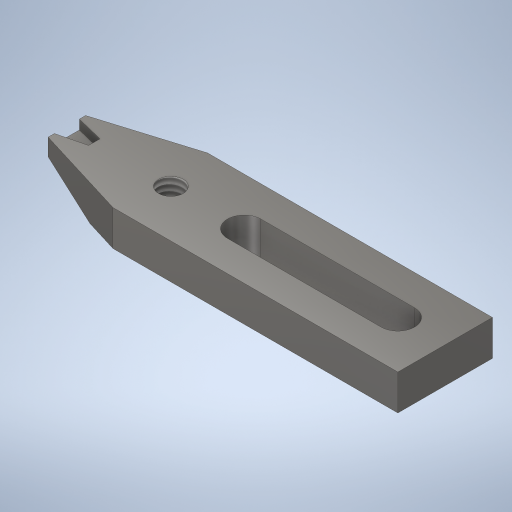
# Autodesk Inventor part: ArmBar-V03- Axel lab
Saved by Autodesk Inventor 2024 (Build 280153000, 153)
## iProperties
Created: 2018-09-07
Part Number: ArmBar-V03- Axel lab
Material: Stainless Steel
Document SubType Name: Modeling
Designer: Tanya
Density: 8 g/cm^3
Appearance: Semi-Polished
Author: Tanya
Autodesk Inventor part; units mm, degrees
ref_plane "YZ Plane" through (0, 0, 0) normal (1, 0, 0) x (0, 1, 0)
ref_plane "XZ Plane" through (0, 0, 0) normal (0, 1, 0) x (-1, 0, 0)
ref_plane "XY Plane" through (0, 0, 0) normal (0, 0, 1) x (1, 0, 0)
sketch "Sketch1" plane through (0, 0, 0) normal (0, 1, 0) x (-1, 0, 0)
  line L0 (0, -8.89) -> (0, 8.89) projected
  line L1 (-35.56, 0) -> (35.56, 0) projected
  line L2 (25.4, -6.35) -> (-25.4, -6.35)
  line L3 (-25.4, -6.35) -> (-25.4, 6.35)
  line L4 (-25.4, 6.35) -> (25.4, 6.35)
  line L5 (25.4, 6.35) -> (25.4, -6.35)
  point P0 (0, 0)
  dimension "d0" = 12.7
  dimension "d1" = 6.35
  dimension "d2" = 50.8
  dimension "d3" = 25.4
  constraints: 8 end point, 2 parallel, 1 horizontal, 1 perpendicular
  measures "d0" distance of L2.end L3.end
  measures "d1" distance between parallel lines of L1 L2
  measures "d2" distance of L2.start L2.end
  measures "d3" distance between parallel lines of L0 L5
extrude "Extrusion1" add sketch "Sketch1" along normal blind 4.7625
sketch "Sketch2" plane through (0, 4.7625, 0) normal (0, 1, 0) x (1, 0, 0)
  line L0 (25.4, 6.35) -> (-25.4, 6.35) projected
  line L1 (-25.4, 6.35) -> (-25.4, -6.35) projected
  line L2 (-25.4, -6.35) -> (25.4, -6.35) projected
  line L3 (25.4, -6.35) -> (25.4, 6.35) projected
  line L4 (-25.4, 2.5146) -> (-12.855, 6.35)
  line L5 (25.4, 6.35) -> (-25.4, 6.35) projected
  line L6 (-25.4, 6.35) -> (-25.4, -6.35) projected
  line L7 (-25.4, -2.5146) -> (-12.855, -6.35)
  line L8 (-12.855, 6.35) -> (-12.855, -6.35) construction
  line L9 (0, 8.89) -> (0, -8.89) projected
  line L10 (35.56, 0) -> (-35.56, 0) projected
  line L11 (-1.5875, 2.2479) -> (19.05, 2.2479)
  line L12 (19.05, 2.2479) -> (19.05, -2.2479)
  line L13 (19.05, -2.2479) -> (-1.5875, -2.2479)
  line L14 (-1.5875, -2.2479) -> (-1.5875, 2.2479)
  circle A0 centre (19.05, 0) radius 2.2479
  circle A1 centre (-1.5875, 0) radius 2.2479
  point P0 (0, 0)
  dimension "d6" = 163
  dimension "d7" = 163
  dimension "d8" = 5.0292
  dimension "d9" = 4.4958
  dimension "d10" = 6.35
  dimension "d11" = 20.6375
  constraints: 14 end point, 7 point on line, 3 parallel, 2 midpoint, 1 centre point, 1 horizontal, 1 perpendicular, 1 tangent, 1 vertical alignment, 2 other
  measures "d6" angle of L0 L4
  measures "d7" angle of L2 L7
  measures "d8" distance of L7.start L4.start
  measures "d9" distance between parallel lines of L13 L11
  measures "d10" distance between parallel lines of L12 L3
  measures "d11" distance of L11.start L11.end
extrude "Extrusion2" cut sketch "Sketch2" against normal through all contours L4 L1 L0 | L11 A0 L10 A1 L9 | L9 A1 L11 | A1 L10 L9 | L9 L10 L14 A1 | L14 L10 A1 | A0 L10 L12 | L12 L10 A0 | L7 L2 L1 | L10 L14 A1 | A0 L12 L10 | L10 A1 L9 | L9 A1 L14 L10 | L10 A0 L13 L9 A1 | L12 A0 L10 | A1 L9 L13
sketch "Sketch3" plane through (0, 4.7625, 0) normal (0, 1, 0) x (1, 0, 0)
  line L0 (-25.4, -2.5146) -> (-12.855, -6.35) projected
  line L1 (-12.855, -6.35) -> (25.4, -6.35) projected
  line L2 (25.4, -6.35) -> (25.4, 6.35) projected
  line L3 (25.4, 6.35) -> (-12.855, 6.35) projected
  line L4 (-12.855, 6.35) -> (-25.4, 2.5146) projected
  line L5 (-25.4, 2.5146) -> (-25.4, -2.5146) projected
  line L6 (19.05, -2.2479) -> (-1.5875, -2.2479) projected
  arc A0 (-1.5875, 2.2479) -> (-1.5875, -2.2479) centre (-1.5875, 0) ccw projected
  line L7 (-1.5875, 2.2479) -> (19.05, 2.2479) projected
  arc A1 (19.05, -2.2479) -> (19.05, 2.2479) centre (19.05, 0) ccw projected
  line L8 (35.56, 0) -> (-35.56, 0) projected
  line L9 (-25.4, 1.6803) -> (-21.717, 0.762)
  line L10 (-21.717, 0.762) -> (-21.717, -0.762)
  line L11 (-21.717, -0.762) -> (-25.4, -1.6803)
  line L12 (-25.4, 2.5146) -> (-25.4, -2.5146) projected
  line L13 (-25.4, 1.6803) -> (-25.4, -1.6803)
  point P0 (0, 0)
  dimension "d14" = 28
  dimension "d15" = 14
  dimension "d16" = 3.683
  dimension "d17" = 1.524
  dimension "d18" = 0.762
  constraints: 8 end point, 2 point on line, 1 perpendicular, 1 vertical
  measures "d14" angle of L11 L9
  measures "d15" angle of L8 L9
  measures "d16" distance between parallel lines of L5 L10
  measures "d17" distance of L9.end L10.end
  measures "d18" distance from line of L8 L9.end
extrude "Extrusion3" cut sketch "Sketch3" against normal blind 1.27 contours L5 L8 L10 L11 | L5 L9 L10 L8
sketch "Sketch4" plane through (0, 4.7625, 0) normal (0, 1, 0) x (1, 0, 0)
  line L0 (19.05, -2.2479) -> (-1.5875, -2.2479) projected
  arc A0 (-1.5875, 2.2479) -> (-1.5875, -2.2479) centre (-1.5875, 0) ccw projected
  line L1 (-1.5875, 2.2479) -> (19.05, 2.2479) projected
  arc A1 (19.05, -2.2479) -> (19.05, 2.2479) centre (19.05, 0) ccw projected
  line L2 (-25.4, 1.6803) -> (-21.717, 0.762) projected
  line L3 (-21.717, 0.762) -> (-21.717, -0.762) projected
  line L4 (-21.717, -0.762) -> (-25.4, -1.6803) projected
  line L5 (-25.4, -1.6803) -> (-25.4, -2.5146) projected
  line L6 (-25.4, -2.5146) -> (-12.855, -6.35) projected
  line L7 (-12.855, -6.35) -> (25.4, -6.35) projected
  line L8 (25.4, -6.35) -> (25.4, 6.35) projected
  line L9 (25.4, 6.35) -> (-12.855, 6.35) projected
  line L10 (-12.855, 6.35) -> (-25.4, 2.5146) projected
  line L11 (-25.4, 2.5146) -> (-25.4, 1.6803) projected
  line L12 (0, 8.89) -> (0, -8.89) projected
  line L13 (35.56, 0) -> (-35.56, 0) projected
  point P0 (0, 0)
  point P1 (-11.43, 0)
  dimension "d21" = 36.83
  constraints: 1 point on line
  measures "d21" distance from line of point (-11.43, 0) L8
hole "Hole1" at (-11.43, 4.7625, 0) direction (0, -1, 0) diameter 3.302 depth 12.2936 tip angle 118 thread size "8-32 UNC" class "2B" standard "ANSI Unified Screw Threads"
sketch "Sketch6" plane through (25.4, 0, 6.35) normal (0, 0, 1) x (1, 0, 0)
  line L0 (-38.255, 0) -> (-50.8, 0) projected
  line L1 (-38.255, 4.7625) -> (-38.255, 0) projected
  line L2 (-50.8, 4.7625) -> (-38.255, 4.7625) projected
  line L3 (-50.8, 0) -> (-50.8, 4.7625) projected
  line L4 (-38.255, 4.7625) -> (-38.255, 0) projected
  line L5 (0, 0) -> (-38.255, 0) projected
  line L6 (0, 0) -> (0, 4.7625) projected
  line L7 (-38.255, 4.7625) -> (0, 4.7625) projected
  line L8 (-50.8, 2.4765) -> (-42.6997, 0)
  line L9 (-50.8, 2.4765) -> (-50.8, -12.0091)
  line L10 (-50.8, -12.0091) -> (-42.6997, -12.0091)
  line L11 (-42.6997, -12.0091) -> (-42.6997, 0)
  point P0 (-25.4, 0)
  dimension "d31" = 163
  dimension "d32" = 2.286
  constraints: 8 end point, 2 point on line, 1 parallel, 1 perpendicular, 1 vertical
  measures "d31" angle of L5 L8
  measures "d32" distance from line of L8.start L2
extrude "Extrusion4" cut sketch "Sketch6" against normal through all contours L11 L10 L9 L0 | L0 L3 L8
equation "\"d1\" = 0.5 * d0"
equation "\"d3\" = 0.5 * d2"
equation "\"d7\" = d6"
equation "\"d15\" = 0.5 * d14"
equation "\"d18\" = 0.5 * d17"
body "Solid1"
